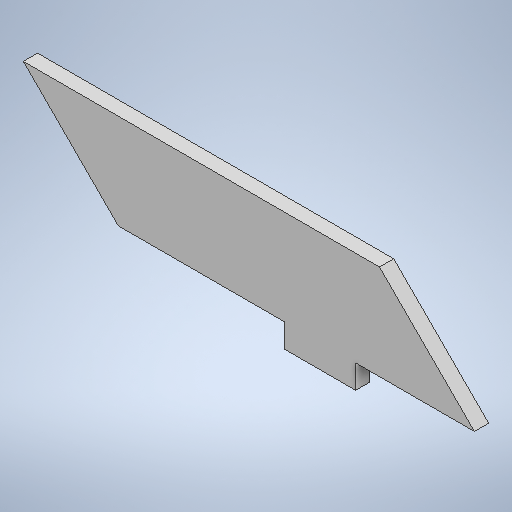
# Autodesk Inventor part: Hinge Siderail 1
Saved by Autodesk Inventor 2025.1 (Build 291241020, 241B)
## iProperties
Created: 2024-10-28
Part Number: Hinge Siderail 1
Material: Generic
Document SubType Name: Modeling
Designer: aly_g
Density: 1 g/cm^3
Appearance: Default
Author: aly_g
Autodesk Inventor part; units mm, degrees
ref_plane "YZ Plane" through (0, 0, 0) normal (1, 0, 0) x (0, 1, 0)
ref_plane "XZ Plane" through (0, 0, 0) normal (0, 1, 0) x (-1, 0, 0)
ref_plane "XY Plane" through (0, 0, 0) normal (0, 0, 1) x (1, 0, 0)
sketch "Sketch1" plane through (0, 0, 0) normal (0, 0, 1) x (1, 0, 0)
  line L0 (0, 0) -> (75, 0)
  line L1 (35, 0) -> (50, 0)
  line L2 (50, 0) -> (50, -5)
  line L3 (50, -5) -> (35, -5)
  line L4 (35, -5) -> (35, 0)
  line L5 (0, 0) -> (-20, 20)
  line L6 (-20, 20) -> (55, 20)
  line L7 (55, 20) -> (75, 0)
  point P0 (50, 0)
  dimension "d0" = 75
  dimension "d3" = 15
  dimension "d4" = 5
  dimension "d5" = 35
  dimension "d19" = 20
  dimension "d20" = 20
  constraints: 16 end point, 3 horizontal, 3 parallel, 1 perpendicular, 1 point on line
  measures "d0" distance of L0.start L0.end
  measures "d3" distance of L2.end L3.end
  measures "d4" distance of L1.start L3.end
  measures "d5" distance of L1.start L0.start
  measures "d19" horizontal distance of L0.start L5.end
  measures "d20" horizontal distance of L0.start L5.end
extrude "Extrusion1" add sketch "Sketch1" along normal blind 3
body "Solid1"
